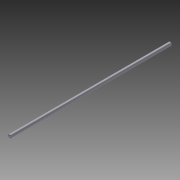
# Autodesk Inventor part: am-0756
Saved by Autodesk Inventor 2011 SP1 (Build 150282100, 282)
## iProperties
Category: Chassis
Company: Autodesk Inc.
Created: 2011-01-10
Part Number: am-0756
Document SubType Name: Modeling
Designer: Autodesk Inc.
Density: 2.71 g/cm^3
Catalog Web Link: http://www.andymark.com/productdetails.asp?productcode=am-0756
Description: Extruded Aluminum Tube, hex profile
Vendor: Andy Mark Inc.
Material: Aluminum-6061
Mass: 203.237 g
Surface Area: 425.337 cm^2
Volume: 74.9953 cm^3
Author: Autodesk Inc.
Autodesk Inventor part; units mm, degrees
ref_plane "YZ Plane" through (0, 0, 0) normal (1, 0, 0) x (0, 1, 0)
ref_plane "XZ Plane" through (0, 0, 0) normal (0, 1, 0) x (-1, 0, 0)
ref_plane "XY Plane" through (0, 0, 0) normal (0, 0, 1) x (1, 0, 0)
sketch "Sketch1" plane through (0, 0, 0) normal (0, 0, 1) x (1, 0, 0)
  circle A0 centre (0, 0) radius 2.9337
  line L0 (3.6295, 6.2865) -> (7.259, 0)
  line L1 (7.259, 0) -> (3.6295, -6.2865)
  line L2 (3.6295, -6.2865) -> (-3.6295, -6.2865)
  line L3 (-3.6295, -6.2865) -> (-7.259, 0)
  line L4 (-7.259, 0) -> (-3.6295, 6.2865)
  line L5 (-3.6295, 6.2865) -> (3.6295, 6.2865)
  dimension "d0" = 5.8674
  dimension "d1" = 12.573
  constraints: 12 end point, 2 coincident, 1 centre point, 13 other
  measures "d0" diameter of A0
  measures "d1" distance between parallel lines of L2 L5
extrude "Extrusion1" add sketch "Sketch1" against normal blind 682.625
body "Solid1"
